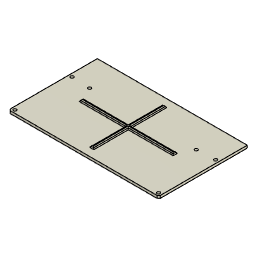
Half Carry Lid (Autodesk Fusion 360 design; units mm, degrees)
Autodesk Fusion 360 part; units mm, degrees
ref_plane "WorkPlane1" through (0, 0, 123.8) normal (0, 0, 1) x (1, 0, 0)
sketch "Sketch1" plane through (0, 0, 123.8) normal (0, 0, 1) x (1, 0, 0)
  circle A0 centre (-85.5, 170) radius 1.4 construction
  line L0 (-81.5, 4) -> (-81.5, 166) construction
  line L1 (-81.5, 166) -> (-81.5, 167) construction
  line L2 (-81.5, 167) -> (-77.5, 167) construction
  line L3 (-77.5, 167) -> (-77.5, 174) construction
  line L4 (-77.5, 174) -> (-81.5, 174) construction
  line L5 (-81.5, 174) -> (-86.5, 174) construction
  line L6 (-87.2574, 174) -> (-87.5, 174) construction
  line L7 (-87.5, 174) -> (-89.5, 172) construction
  line L8 (-89.5, 172) -> (-89.5, 0) construction
  line L9 (-89.5, 0) -> (-81.5, 0) construction
  line L10 (-81.5, 0) -> (-81.5, 4) construction
  circle A1 centre (85.5, 170) radius 1.4 construction
  line L11 (89.5, 0) -> (89.5, 172) construction
  line L12 (89.5, 172) -> (87.5, 174) construction
  line L13 (87.5, 174) -> (86.5, 174) construction
  line L14 (86.5, 174) -> (86.5, 177) construction
  line L15 (86.5, 177) -> (86.45, 177) construction
  line L16 (86.45, 177) -> (86.45, 174) construction
  line L17 (86.45, 174) -> (81.5, 174) construction
  line L18 (81.5, 174) -> (77.5, 174) construction
  line L19 (77.5, 174) -> (77.5, 167) construction
  line L20 (77.5, 167) -> (81.5, 167) construction
  line L21 (81.5, 167) -> (81.5, 0) construction
  line L22 (81.5, 0) -> (89.5, 0) construction
  line L23 (81.5, 0) -> (81.5, -37.7937) construction
  line L24 (81.5, -37.7937) -> (87.5, -37.7937) construction
  line L25 (87.5, -37.7937) -> (89.5, -35.7937) construction
  line L26 (89.5, -35.7937) -> (89.5, -5) construction
  line L27 (89.5, -5) -> (89.5, 0) construction
  line L28 (89.5, 0) -> (81.5, 0) construction
  line L29 (-89.5, 0) -> (-89.5, -35.7937) construction
  line L30 (-89.5, -35.7937) -> (-87.5, -37.7937) construction
  line L31 (-87.5, -37.7937) -> (-81.5, -37.7937) construction
  line L32 (-81.5, -37.7937) -> (-81.5, -5) construction
  line L33 (-81.5, -5) -> (-81.5, 0) construction
  line L34 (-81.5, 0) -> (-89.5, 0) construction
  line L35 (87.5, -37.7937) -> (-87.5, -37.7937) construction
  line L36 (-77.3, 174) -> (77.3, 174) construction
  line L37 (-77.5, 174) -> (77.5, 174)
  line L38 (77.5, 174) -> (87.5, 174)
  line L39 (87.5, 174) -> (89.5, 172)
  line L40 (89.5, 172) -> (89.5, -35.7937)
  line L41 (89.5, -35.7937) -> (87.5, -37.7937)
  line L42 (-87.5, -37.7937) -> (87.5, -37.7937)
  line L43 (-87.5, -37.7937) -> (-89.5, -35.7937)
  line L44 (-89.5, -35.7937) -> (-89.5, 172)
  line L45 (-89.5, 172) -> (-87.5, 174)
  line L46 (-87.5, 174) -> (-77.3, 174)
  circle A2 centre (-85.5, 170) radius 1.8
  circle A3 centre (-85.5, 102) radius 1.8
  circle A4 centre (-85.5, 34) radius 1.8
  circle A5 centre (-85.5, -34) radius 1.8
  circle A6 centre (85.5, -34) radius 1.8
  circle A7 centre (85.5, 34) radius 1.8
  circle A8 centre (85.5, 102) radius 1.8
  circle A9 centre (85.5, 170) radius 1.8
  line L47 (-86.5, 174) -> (-87.2574, 174)
  circle A10 centre (85.5, -34) radius 1.4 construction
  circle A11 centre (-85.5, -34) radius 1.4 construction
  circle A12 centre (-85.5, 34) radius 1.4 construction
  circle A13 centre (-85.5, 102) radius 1.4 construction
  circle A14 centre (85.5, 102) radius 1.4 construction
  circle A15 centre (85.5, 34) radius 1.4 construction
  line L48 (-89.5, 68.1031) -> (89.5, 68.1031) construction
  line L49 (-89.5, 67.9531) -> (89.5, 67.9531)
  line L50 (-77.5, 173.8) -> (-77.3, 173.8)
  line L51 (-77.3, 173.8) -> (77.5, 173.8)
  line L52 (77.5, 173.8) -> (87.4172, 173.8)
  line L53 (87.4172, 173.8) -> (89.3, 171.9172)
  line L54 (89.3, 171.9172) -> (89.3, -35.7109)
  line L55 (89.3, -35.7109) -> (87.4172, -37.5937)
  line L56 (-87.4172, -37.5937) -> (87.4172, -37.5937)
  line L57 (-87.4172, -37.5937) -> (-89.3, -35.7109)
  line L58 (-89.3, -35.7109) -> (-89.3, 171.9172)
  line L59 (-89.3, 171.9172) -> (-87.4172, 173.8)
  line L60 (-87.4172, 173.8) -> (-77.3, 173.8)
  dimension "d2" = 0.2
  dimension "d4" = 3.6
  dimension "d5" = 3.6
  dimension "d6" = 3.6
  dimension "d7" = 3.6
  dimension "d8" = 3.6
  dimension "d9" = 3.6
  dimension "d10" = 3.6
  dimension "d11" = 3.6
  dimension "d14" = 0.15
  constraint coincident L3.end L4.start
  constraint coincident L18.end L19.start
  constraint coincident L12.end L13.start
  constraint coincident L11.end L12.start
  constraint coincident L25.end L26.start
  constraint coincident L24.end L25.start
  constraint coincident L30.end L31.start
  constraint coincident L29.end L30.start
  constraint coincident L7.end L8.start
  constraint coincident L6.end L7.start
  constraint coincident L36.start L46.end
  constraint concentric A0 A2
  constraint concentric A1 A9
  constraint concentric A6 A10
  constraint concentric A5 A11
  constraint concentric A4 A12
  constraint concentric A7 A15
  constraint concentric A8 A14
  constraint concentric A3 A13
  constraint midpoint L44 L48.start
  constraint midpoint L40 L48.end
  measures "d4" diameter of A2
  measures "d5" diameter of A9
  measures "d6" diameter of A8
  measures "d7" diameter of A3
  measures "d8" diameter of A7
  measures "d9" diameter of A6
  measures "d10" diameter of A4
  measures "d11" diameter of A5
extrude "Extrude1" add sketch "Sketch1" along normal blind 3 contours L49 L54 L55 L56 L57 L58
sketch "Sketch2" plane through (0, 0, 126.8) normal (0, 0, 1) x (-1, 0, 0)
  circle A0 centre (85.5, 34) radius 1.8
  circle A1 centre (-85.5, 34) radius 1.8
  circle A2 centre (-85.5, -34) radius 1.8
  circle A3 centre (85.5, -34) radius 1.8
  line L0 (87.4172, 37.5937) -> (-87.4172, 37.5937)
  line L1 (-87.4172, 37.5937) -> (-89.3, 35.7109)
  line L2 (-89.3, 35.7109) -> (-89.3, -67.9531)
  line L3 (-89.3, -67.9531) -> (89.3, -67.9531)
  line L4 (89.3, -67.9531) -> (89.3, 35.7109)
  line L5 (89.3, 35.7109) -> (87.4172, 37.5937)
  line L6 (0, -67.9531) -> (0, 37.5937) construction
  line L7 (0, -67.9531) -> (0, -32.9531) construction
  line L8 (0, -32.9531) -> (-63.5, -32.9531) construction
  circle A4 centre (-63.5, -32.9531) radius 1.8
  circle A5 centre (63.5, -32.9531) radius 1.8
  dimension "d15" = 35
  dimension "d16" = 63.5
  dimension "d17" = 3.6
  constraint midpoint L3 L6.start
  constraint midpoint L0 L6.end
  constraint perpendicular L0 L7
  constraint perpendicular L6 L8
  constraint coincident L8.end A4.centre
  constraint symmetric L6 A4 A5
  measures "d15" distance of L6.start L7.end
  measures "d16" distance of L7.end L8.end
  measures "d17" diameter of A4
extrude "Extrude2" cut sketch "Sketch2" against normal blind 3 contours A4 | A5
sketch "Sketch3" plane through (0, 0, 126.8) normal (0, 0, 1) x (-1, 0, 0)
  circle A0 centre (-63.5, -32.9531) radius 1.8
  circle A1 centre (63.5, -32.9531) radius 1.8
  circle A2 centre (85.5, 34) radius 1.8
  circle A3 centre (-85.5, 34) radius 1.8
  circle A4 centre (-85.5, -34) radius 1.8
  circle A5 centre (85.5, -34) radius 1.8
  line L0 (87.4172, 37.5937) -> (-87.4172, 37.5937)
  line L1 (-87.4172, 37.5937) -> (-89.3, 35.7109)
  line L2 (-89.3, 35.7109) -> (-89.3, -67.9531)
  line L3 (-89.3, -67.9531) -> (89.3, -67.9531)
  line L4 (89.3, -67.9531) -> (89.3, 35.7109)
  line L5 (89.3, 35.7109) -> (87.4172, 37.5937)
  line L6 (0, -67.9531) -> (0, -57.9531) construction
  line L7 (0, -57.9531) -> (0, 27.0469) construction
  line L8 (0, -15.4531) -> (-55, -15.4531) construction
  line L9 (0, -15.4531) -> (55, -15.4531) construction
  line L10 (1.5, -13.9531) -> (55, -13.9531)
  line L11 (-1.5, -13.9531) -> (-55, -13.9531)
  line L12 (1.5, -16.9531) -> (55, -16.9531)
  line L13 (-1.5, -16.9531) -> (-55, -16.9531)
  line L14 (-55, -16.9531) -> (-55, -13.9531)
  line L15 (55, -16.9531) -> (55, -13.9531)
  line L16 (-1.5, -57.9531) -> (1.5, -57.9531)
  line L17 (1.5, 27.0469) -> (-1.5, 27.0469)
  line L18 (1.5, -57.9531) -> (1.5, -16.9531)
  line L19 (1.5, -13.9531) -> (1.5, 27.0469)
  line L20 (-1.5, -57.9531) -> (-1.5, -16.9531)
  line L21 (-1.5, -13.9531) -> (-1.5, 27.0469)
  dimension "d20" = 10
  dimension "d21" = 85
  dimension "d22" = 55
  dimension "d23" = 55
  constraint midpoint L3 L6.start
  constraint perpendicular L0 L6
  constraint perpendicular L0 L7
  constraint midpoint L7 L8.start
  constraint perpendicular L7 L8
  constraint perpendicular L7 L9
  constraint perpendicular L11 L14
  constraint perpendicular L10 L15
  constraint perpendicular L16 L18
  constraint parallel L7 L20
  constraint perpendicular L17 L20
  constraint parallel L9 L10
  constraint parallel L8 L11
  constraint coincident L10.start L18
  constraint parallel L7 L18
  constraint collinear L18 L19
  constraint parallel L9 L12
  constraint parallel L8 L13
  constraint coincident L11.start L20
  constraint collinear L20 L21
  measures "d20" distance of L6.start L6.end
  measures "d21" distance of L6.end L7.end
  measures "d22" distance of L8.start L8.end
  measures "d23" distance of L8.start L9.end
extrude "Extrude3" add sketch "Sketch3" along normal blind 2 contours L10 L11 L12 L13 L14 L15 L16 L17 L18 L19 L20 L21
fillet "Fillet1" radius 1 12 edges at (-28.25, 13.9531, 126.8) (-1.5, -6.5469, 126.8) (-55, 15.4531, 126.8) (0, -27.0469, 126.8) (1.5, -6.5469, 126.8) (28.25, 13.9531, 126.8) (1.5, 37.4531, 126.8) (55, 15.4531, 126.8) (28.25, 16.9531, 126.8) (0, 57.9531, 126.8) (-28.25, 16.9531, 126.8) (-1.5, 37.4531, 126.8) 1 faces at (19.3333, 15.9531, 128.8)
equation "large_m3 = 3.6 mm"
equation "d4 = large_m3"
equation "d5 = d4"
equation "d6 = d4"
equation "d7 = d4"
equation "d8 = d4"
equation "d9 = d4"
equation "d10 = d4"
equation "d11 = d4"
equation "d16 = ( 127 / 2 ) * 1 mm"
